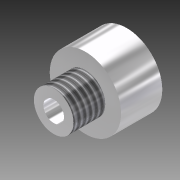
# Autodesk Inventor part: 1in Actuator Top Cap 1764
Saved by Autodesk Inventor 2011 (Build 150239000, 239)
## iProperties
Created: 2010-02-07
Part Number: 1in Actuator Top Cap 1764
Document SubType Name: Modeling
Designer: jgehrig
Density: 1 g/cm^3
Author: jgehrig
Autodesk Inventor part; units mm, degrees
ref_plane "YZ Plane" through (0, 0, 0) normal (1, 0, 0) x (0, 1, 0)
ref_plane "XY Plane" through (0, 0, 0) normal (0, 0, 1) x (1, 0, 0)
sketch "Sketch1" plane through (0, 0, 0) normal (0, 0, 1) x (1, 0, 0)
  circle A0 centre (0, 0) radius 14.2875
  circle A1 centre (0, 0) radius 12.065
  dimension "d0" = 28.575
  dimension "d1" = 24.13
  constraints: 2 centre point, 2 coincident
  measures "d0" diameter of A0
  measures "d1" diameter of A1
extrude "Extrusion1" add sketch "Sketch1" along normal blind 13.97
sketch "Sketch2" plane through (0, 0, 13.97) normal (0, 0, 1) x (1, 0, 0)
  circle A0 centre (0, 0) radius 14.2875 projected
  circle A1 centre (0, 0) radius 14.2875
  constraints: 1 centre point, 1 coincident, 1 concentric
extrude "Extrusion2" add sketch "Sketch2" along normal blind 2.54
sketch "Sketch3" plane through (0, 0, 16.51) normal (0, 0, 1) x (1, 0, 0)
  circle A0 centre (0, 0) radius 14.2875 projected
  circle A1 centre (0, 0) radius 7.9375
  dimension "d6" = 15.875
  constraints: 1 centre point, 1 coincident
  measures "d6" diameter of A1
extrude "Extrusion3" add sketch "Sketch3" along normal blind 12.7 contours A1
thread "Thread1" size "5/8-11 UNC" class "2A" standard "ANSI Unified Screw Threads" full length
ref_plane "Work Plane1" through (0, -14.2875, 0) normal (0, 1, 0) x (-1, 0, 0)
sketch "Sketch4" plane through (0, -14.2875, 0) normal (0, 1, 0) x (-1, 0, 0)
  line L0 (-14.2875, 16.51) -> (14.2875, 16.51) projected
  line L1 (-14.2875, 0) -> (14.2875, 0) projected
  circle A0 centre (0, 8.255) radius 5.3975
  point P0 (0, 0)
  dimension "d12" = 10.795
  dimension "d13" = 8.255
  constraints: 1 centre point
  measures "d12" diameter of A0
  measures "d13" distance from line of L0 A0.centre
extrude "Extrusion4" cut sketch "Sketch4" along normal blind 12.7
sketch "Sketch5" plane through (0, 0, 29.21) normal (0, 0, 1) x (1, 0, 0)
  circle A0 centre (0, 0) radius 7.9375 projected
  circle A1 centre (0, 0) radius 4.1275
  dimension "d16" = 8.255
  constraints: 1 centre point, 1 coincident
  measures "d16" diameter of A1
extrude "Extrusion5" cut sketch "Sketch5" against normal through all contours A1
body "Solid1"
